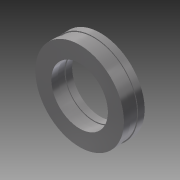
# Autodesk Inventor part: Thrust Bearing 51106 - 30x47x11mm
Saved by Autodesk Inventor 2013 (Build 170138000, 138)
## iProperties
Created: 2014-10-12
Part Number: Thrust Bearing 51106 - 30x47x11mm
Material: Stainless Steel
Document SubType Name: Modeling
Designer: Masta
Density: 1 g/cm^3
Author: Masta
Autodesk Inventor part; units mm, degrees
ref_plane "YZ Plane" through (0, 0, 0) normal (1, 0, 0) x (0, 1, 0)
ref_plane "XZ Plane" through (0, 0, 0) normal (0, 1, 0) x (-1, 0, 0)
ref_plane "XY Plane" through (0, 0, 0) normal (0, 0, 1) x (1, 0, 0)
sketch "Sketch1" plane through (0, 0, 0) normal (0, 1, 0) x (-1, 0, 0)
  circle A0 centre (0, 0) radius 15
  circle A1 centre (0, 0) radius 23.5
  circle A2 centre (0, 0) radius 15.5
  circle A3 centre (0, 0) radius 23
  dimension "d0" = 30
  dimension "d1" = 47
  dimension "d2" = 0.5
  dimension "d3" = 0.5
  constraints: 4 centre point, 4 coincident
  measures "d0" diameter of A0
  measures "d1" diameter of A1
  measures "d2" radial gap between concentric circles of A1 A3
  measures "d3" radial gap between concentric circles of A0 A2
extrude "Extrusion1" add sketch "Sketch1" along normal mid plane 11 contours A1 | A2 | A3
extrude "Extrusion2" cut sketch "Sketch1" along normal mid plane 4
body "Solid1"
